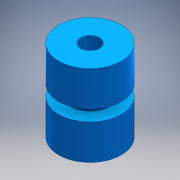
# Autodesk Inventor part: roller
Saved by Autodesk Inventor 2016 (Build 200138000, 138)
## iProperties
Created: 2016-05-25
Part Number: roller
Material: ABS Plastic
Document SubType Name: Modeling
Designer: Henrik Samuelsson
Density: 1.06 g/cm^3
Appearance: Smooth - White
Author: Henrik Samuelsson
Autodesk Inventor part; units mm, degrees
ref_plane "YZ Plane" through (0, 0, 0) normal (1, 0, 0) x (0, 1, 0)
ref_plane "XZ Plane" through (0, 0, 0) normal (0, 1, 0) x (-1, 0, 0)
ref_plane "XY Plane" through (0, 0, 0) normal (0, 0, 1) x (1, 0, 0)
sketch "Sketch1" plane through (0, 0, 0) normal (0, 1, 0) x (-1, 0, 0)
  line L0 (0, 0) -> (0, -2.5)
  line L1 (3.5, 0.5) -> (0, 0)
  line L2 (3.5, -3) -> (0, -2.5)
  line L3 (3.5, -3) -> (3.5, -14.25)
  line L4 (3.5, -14.25) -> (-6.5, -14.25)
  line L5 (3.5, 0.5) -> (3.5, 11.75)
  line L6 (3.5, 11.75) -> (-6.5, 11.75)
  line L7 (-6.5, 11.75) -> (-6.5, -14.25)
  dimension "d0" = 2.5
  dimension "d6" = 3.5
  dimension "d9" = 11.25
  dimension "d11" = 10
  dimension "d12" = 90
  dimension "d13" = 11.25
  dimension "d15" = 10
  dimension "d16" = 90
  dimension "d17" = 3.5
  dimension "d18" = 11.75
  constraints: 16 end point, 3 perpendicular, 3 vertical
  measures "d0" distance of L0.start L0.end
  measures "d6" horizontal distance of L0.start L1.start
  measures "d9" distance of L2.start L3.end
  measures "d11" distance of L3.end L4.end
  measures "d12" angle of L3 L4
  measures "d13" distance of L1.start L5.end
  measures "d15" distance of L5.end L6.end
  measures "d16" angle of L6 L5
  measures "d17" distance of L2.start L1.start
  measures "d18" distance from line of L0.start L6
revolve "Revolution1" add sketch "Sketch1" angle 360 about axis through (6.5, 0, 11.75) along (0, 0, -1)
sketch "Sketch2" plane through (6.5, 0, -14.25) normal (0, 0, -1) x (-1, 0, 0)
  circle A0 centre (0, 0) radius 3
  circle A1 centre (0, 0) radius 10 projected
  point P0 (6.5, 0)
  dimension "d20" = 6
  constraints: 1 centre point, 1 concentric
  measures "d20" diameter of A0
extrude "Extrusion1" cut sketch "Sketch2" against normal blind 26 contours A0
body "Solid1"
